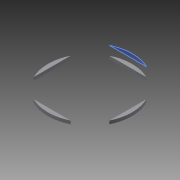
# Autodesk Inventor part: snap
Saved by Autodesk Inventor 2014 (Build 180170000, 170)
## iProperties
Created: 2013-05-26
Part Number: snap
Material: Generisch
Document SubType Name: Modeling
Designer: Felix
Density: 1 g/cm^3
Appearance: Vorgabe
Author: Felix
Autodesk Inventor part; units mm, degrees
ref_plane "YZ Plane" through (0, 0, 0) normal (1, 0, 0) x (0, 1, 0)
ref_plane "XZ Plane" through (0, 0, 0) normal (0, 1, 0) x (-1, 0, 0)
ref_plane "XY Plane" through (0, 0, 0) normal (0, 0, 1) x (1, 0, 0)
sketch "Sketch1" plane through (0, 0, 0) normal (0, 0, 1) x (1, 0, 0)
  circle A0 centre (0, 0) radius 11.0482 projected
  circle A1 centre (0, 0) radius 13.0482 projected
  line L0 (-5.7202, 11.7276) -> (5.7202, 11.7276)
  line L1 (11.7276, 5.7202) -> (11.7276, -5.7202)
  line L2 (5.7202, -11.7276) -> (-5.7202, -11.7276)
  line L3 (-11.7276, 5.7202) -> (-11.7276, -5.7202)
  point P0 (0, 0)
  constraints: 8 end point, 3 equal length, 3 perpendicular, 1 horizontal, 9 other
extrude "Extrusion1" add sketch "Sketch1" along normal blind 1 contours A1 L1 | L0 A1 | A1 L2 | L3 A1
body "Solid1"
